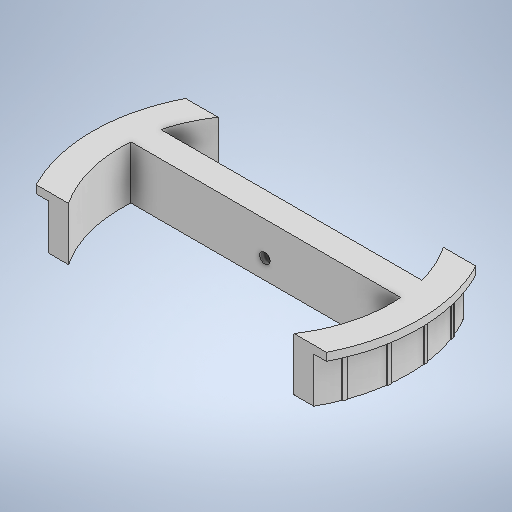
# Autodesk Inventor part: Part6
Saved by Autodesk Inventor 2025 (Build 290162010, 162A)
## iProperties
Created: 2024-07-08
Part Number: Part6
Material: Generic
Document SubType Name: Modeling
Designer: vncnt
Density: 1 g/cm^3
Appearance: Default
Author: vncnt
## iProperties of the stored document AQS_Mount_3DPrint.ipt
Created: 2024-07-08
Part Number: AQS_Mount_3DPrint
Material: Generic
Document SubType Name: Modeling
Designer: vncnt
Density: 1 g/cm^3
Appearance: Default
Author: vncnt
Autodesk Inventor part; units mm, degrees
ref_plane "YZ Plane" through (0, 0, 0) normal (1, 0, 0) x (0, 1, 0)
ref_plane "XZ Plane" through (0, 0, 0) normal (0, 1, 0) x (-1, 0, 0)
ref_plane "XY Plane" through (0, 0, 0) normal (0, 0, 1) x (1, 0, 0)
sketch "Sketch1" plane through (0, 0, 0) normal (0, 1, 0) x (-1, 0, 0)
  line L0 (33.8585, -6) -> (-33.8585, -6)
  line L1 (-34.295, -2.5) -> (34.295, -2.5)
  line L2 (0.5017, -38.45) -> (-0.4983, -38.45)
  line L3 (-0.4983, -38.45) -> (-0.4983, -38.85)
  line L4 (-0.4983, -38.85) -> (0.5017, -38.85)
  line L5 (0.5017, -38.85) -> (0.5017, -38.45)
  line L6 (0.5017, -38.45) -> (-0.4983, -38.85) construction
  line L7 (-0.4983, -38.45) -> (0.5017, -38.85) construction
  line L8 (9.6888, -37.2126) -> (8.7179, -37.452)
  line L9 (8.7179, -37.452) -> (8.8136, -37.8403)
  line L10 (8.8136, -37.8403) -> (9.7846, -37.601)
  line L11 (9.7846, -37.601) -> (9.6888, -37.2126)
  line L12 (18.3129, -33.8126) -> (17.4274, -34.2773)
  line L13 (17.4274, -34.2773) -> (17.6133, -34.6315)
  line L14 (17.6133, -34.6315) -> (18.4987, -34.1668)
  line L15 (18.4987, -34.1668) -> (18.3129, -33.8126)
  line L16 (25.8726, -28.4475) -> (25.1241, -29.1107)
  line L17 (25.1241, -29.1107) -> (25.3893, -29.4101)
  line L18 (25.3893, -29.4101) -> (26.1379, -28.7469)
  line L19 (26.1379, -28.7469) -> (25.8726, -28.4475)
  line L20 (31.9287, -21.4292) -> (31.3607, -22.2522)
  line L21 (31.3607, -22.2522) -> (31.6899, -22.4794)
  line L22 (31.6899, -22.4794) -> (32.2579, -21.6564)
  line L23 (32.2579, -21.6564) -> (31.9287, -21.4292)
  line L24 (36.1293, -13.1654) -> (35.7747, -14.1005)
  line L25 (35.7747, -14.1005) -> (36.1487, -14.2423)
  line L26 (36.1487, -14.2423) -> (36.5033, -13.3073)
  line L27 (36.5033, -13.3073) -> (36.1293, -13.1654)
  line L28 (38.2301, -4.1366) -> (38.1096, -5.1293)
  line L29 (38.1096, -5.1293) -> (38.5067, -5.1775)
  line L30 (38.5067, -5.1775) -> (38.6272, -4.1848)
  line L31 (38.6272, -4.1848) -> (38.2301, -4.1366)
  line L32 (38.1092, 5.1327) -> (38.2297, 4.14)
  line L33 (38.2297, 4.14) -> (38.6268, 4.1882)
  line L34 (38.6268, 4.1882) -> (38.5063, 5.1809)
  line L35 (38.5063, 5.1809) -> (38.1092, 5.1327)
  line L36 (35.7735, 14.1037) -> (36.1281, 13.1687)
  line L37 (36.1281, 13.1687) -> (36.5021, 13.3105)
  line L38 (36.5021, 13.3105) -> (36.1475, 14.2455)
  line L39 (36.1475, 14.2455) -> (35.7735, 14.1037)
  line L40 (31.3587, 22.255) -> (31.9268, 21.432)
  line L41 (31.9268, 21.432) -> (32.256, 21.6592)
  line L42 (32.256, 21.6592) -> (31.6879, 22.4822)
  line L43 (31.6879, 22.4822) -> (31.3587, 22.255)
  line L44 (25.1215, 29.1129) -> (25.87, 28.4498)
  line L45 (25.87, 28.4498) -> (26.1353, 28.7492)
  line L46 (26.1353, 28.7492) -> (25.3868, 29.4123)
  line L47 (25.3868, 29.4123) -> (25.1215, 29.1129)
  line L48 (17.4244, 34.2789) -> (18.3098, 33.8142)
  line L49 (18.3098, 33.8142) -> (18.4957, 34.1684)
  line L50 (18.4957, 34.1684) -> (17.6102, 34.6331)
  line L51 (17.6102, 34.6331) -> (17.4244, 34.2789)
  line L52 (8.7145, 37.4528) -> (9.6855, 37.2135)
  line L53 (9.6855, 37.2135) -> (9.7812, 37.6018)
  line L54 (9.7812, 37.6018) -> (8.8103, 37.8412)
  line L55 (8.8103, 37.8412) -> (8.7145, 37.4528)
  line L56 (-0.5017, 38.45) -> (0.4983, 38.45)
  line L57 (0.4983, 38.45) -> (0.4983, 38.85)
  line L58 (0.4983, 38.85) -> (-0.5017, 38.85)
  line L59 (-0.5017, 38.85) -> (-0.5017, 38.45)
  line L60 (-9.6888, 37.2126) -> (-8.7179, 37.452)
  line L61 (-8.7179, 37.452) -> (-8.8136, 37.8403)
  line L62 (-8.8136, 37.8403) -> (-9.7846, 37.601)
  line L63 (-9.7846, 37.601) -> (-9.6888, 37.2126)
  line L64 (-18.3129, 33.8126) -> (-17.4274, 34.2773)
  line L65 (-17.4274, 34.2773) -> (-17.6133, 34.6315)
  line L66 (-17.6133, 34.6315) -> (-18.4987, 34.1668)
  line L67 (-18.4987, 34.1668) -> (-18.3129, 33.8126)
  line L68 (-25.8726, 28.4475) -> (-25.1241, 29.1107)
  line L69 (-25.1241, 29.1107) -> (-25.3893, 29.4101)
  line L70 (-25.3893, 29.4101) -> (-26.1379, 28.7469)
  line L71 (-26.1379, 28.7469) -> (-25.8726, 28.4475)
  line L72 (-31.9287, 21.4292) -> (-31.3607, 22.2522)
  line L73 (-31.3607, 22.2522) -> (-31.6899, 22.4794)
  line L74 (-31.6899, 22.4794) -> (-32.2579, 21.6564)
  line L75 (-32.2579, 21.6564) -> (-31.9287, 21.4292)
  line L76 (-36.1293, 13.1654) -> (-35.7747, 14.1005)
  line L77 (-35.7747, 14.1005) -> (-36.1487, 14.2423)
  line L78 (-36.1487, 14.2423) -> (-36.5033, 13.3073)
  line L79 (-36.5033, 13.3073) -> (-36.1293, 13.1654)
  line L80 (-38.2301, 4.1366) -> (-38.1096, 5.1293)
  line L81 (-38.1096, 5.1293) -> (-38.5067, 5.1775)
  line L82 (-38.5067, 5.1775) -> (-38.6272, 4.1848)
  line L83 (-38.6272, 4.1848) -> (-38.2301, 4.1366)
  line L84 (-38.1092, -5.1327) -> (-38.2297, -4.14)
  line L85 (-38.2297, -4.14) -> (-38.6268, -4.1882)
  line L86 (-38.6268, -4.1882) -> (-38.5063, -5.1809)
  line L87 (-38.5063, -5.1809) -> (-38.1092, -5.1327)
  line L88 (-35.7735, -14.1037) -> (-36.1281, -13.1687)
  line L89 (-36.1281, -13.1687) -> (-36.5021, -13.3105)
  line L90 (-36.5021, -13.3105) -> (-36.1475, -14.2455)
  line L91 (-36.1475, -14.2455) -> (-35.7735, -14.1037)
  line L92 (-31.3587, -22.255) -> (-31.9268, -21.432)
  line L93 (-31.9268, -21.432) -> (-32.256, -21.6592)
  line L94 (-32.256, -21.6592) -> (-31.6879, -22.4822)
  line L95 (-31.6879, -22.4822) -> (-31.3587, -22.255)
  line L96 (-25.1215, -29.1129) -> (-25.87, -28.4498)
  line L97 (-25.87, -28.4498) -> (-26.1353, -28.7492)
  line L98 (-26.1353, -28.7492) -> (-25.3868, -29.4123)
  line L99 (-25.3868, -29.4123) -> (-25.1215, -29.1129)
  line L100 (-17.4244, -34.2789) -> (-18.3098, -33.8142)
  line L101 (-18.3098, -33.8142) -> (-18.4957, -34.1684)
  line L102 (-18.4957, -34.1684) -> (-17.6102, -34.6331)
  line L103 (-17.6102, -34.6331) -> (-17.4244, -34.2789)
  line L104 (-8.7145, -37.4528) -> (-9.6855, -37.2135)
  line L105 (-9.6855, -37.2135) -> (-9.7812, -37.6018)
  line L106 (-9.7812, -37.6018) -> (-8.8103, -37.8412)
  line L107 (-8.8103, -37.8412) -> (-8.7145, -37.4528)
  arc A0 (-33.6574, 19) -> (32.0907, -21.5409) centre (0, 0) ccw
  arc A1 (33.6574, -19) -> (33.6574, 19) centre (0, 0) ccw
  arc A2 (32.0887, 21.5438) -> (-32.0907, 21.5409) centre (0, 0) ccw
  line L108 (36.1642, -3.8857) -> (36.1642, -3.8892)
  line L109 (36.1642, -4.8931) -> (36.1642, -4.8965)
  line L110 (-34.9312, -4.7468) -> (-34.9312, -4.7433)
  line L111 (-34.9312, -3.7395) -> (-34.9312, -3.736)
  line L112 (33.6574, -19) -> (28.66, -19)
  line L113 (-28.66, -19) -> (-33.6574, -19)
  line L114 (-33.6574, 19) -> (-28.66, 19)
  line L115 (28.66, 19) -> (33.6574, 19)
  arc A3 (28.66, -19) -> (33.8585, -6) centre (0, 0) ccw
  arc A4 (34.295, -2.5) -> (28.66, 19) centre (0, 0) ccw
  arc A5 (-28.66, 19) -> (-34.295, -2.5) centre (0, 0) ccw
  arc A6 (-33.8585, -6) -> (-28.66, -19) centre (0, 0) ccw
  point P0 (0.0017, -38.65)
  point P1 (35.9587, -14.1702)
  point P2 (36.3132, -13.2352)
  point P3 (38.3049, -5.153)
  point P4 (38.4254, -4.1603)
  point P5 (38.4251, 4.1637)
  point P6 (38.3045, 5.1564)
  point P7 (36.3121, 13.2384)
  point P8 (35.9574, 14.1734)
  point P9 (-35.9587, 14.1702)
  point P10 (-36.3132, 13.2352)
  point P11 (-38.3049, 5.153)
  point P12 (-38.4254, 4.1603)
  point P13 (-38.4251, -4.1637)
  point P14 (-38.3045, -5.1564)
  point P15 (-36.3121, -13.2384)
  point P16 (-35.9574, -14.1734)
  dimension "d2" = 2.5
  dimension "d3" = 3.5
  dimension "d10" = 1
  dimension "d11" = 0.4
  dimension "d14" = 360
  dimension "d18" = 38.65
  dimension "d19" = 4.9974
  constraints: 232 end point, 16 point on circle, 11 parallel, 11 point on line, 7 centre point, 4 horizontal, 3 perpendicular, 2 midpoint, 1 coincident, 209 other
  measures "d2" distance from line of L1 point (0, 0)
  measures "d3" distance between parallel lines of L1 L0
  measures "d10" distance of L4.end L3.end
  measures "d11" distance of L3.end L2.end
  measures "d18" radius of A0
  measures "d19" distance of L113.start L113.end
extrude "Extrusion1" add sketch "Sketch1" along normal blind 11.5 contours L0 A6 L113 A0 L91 L88 L89 L87 L84 L85 L83 L80 L81 L79 L76 L77 L114 A5 L1 A4 L115 A1 L39 L36 L37 L35 L32 L33 L31 L28 L29 L27 L24 L25 L112 A3 | A1 L27 L26 L25 | L25 L24 L27 A1 | A0 L89 L88 L91 | L91 L90 L89 A0 | A1 L31 L30 L29 | L29 L28 L31 A1 | A0 L85 L84 L87 | L87 L86 L85 A0 | A1 L35 L34 L33 | L33 L32 L35 A1 | A0 L81 L80 L83 | L83 L82 L81 A0 | A1 L39 L38 L37 | L37 L36 L39 A1 | A0 L77 L76 L79 | L79 L78 L77 A0
sketch "Sketch2" plane through (0, 11.5, 0) normal (0, 1, 0) x (1, 0, 0)
  arc A0 (33.8585, 6) -> (28.66, 19) centre (0, 0) ccw projected
  line L0 (34.295, 2.5) -> (-34.295, 2.5)
  line L1 (-3.804, 9) -> (7.0469, 9)
  line L2 (33.1873, 9) -> (-33.1873, 9)
  line L3 (-28.66, 19) -> (-33.6574, 19) projected
  line L4 (-33.6574, -19) -> (-28.66, -19) projected
  line L5 (-28.66, -19) -> (-36.8951, -19)
  arc A1 (-34.295, 2.5) -> (-28.66, -19) centre (0, 0) ccw
  arc A2 (28.66, -19) -> (34.295, 2.5) centre (0, 0) ccw
  arc A3 (36.8951, -19) -> (36.8951, 19) centre (0, 0) ccw
  arc A4 (-36.8951, 19) -> (-36.8951, -19) centre (0, 0) ccw
  arc A5 (33.1873, 9) -> (28.66, 19) centre (0, 0) ccw
  arc A6 (-28.66, 19) -> (-33.1873, 9) centre (0, 0) ccw
  line L6 (36.8951, 19) -> (28.66, 19)
  line L7 (-28.66, 19) -> (-36.8951, 19)
  line L8 (-31.7819, -19) -> (-28.66, -19)
  line L9 (28.66, -19) -> (36.8951, -19)
  line L10 (-30.5962, 19) -> (-28.66, 19)
  line L11 (28.66, 19) -> (36.8951, 19)
  point P0 (28.66, 19)
  point P1 (7.0469, 9)
  dimension "d24" = 41.5
  dimension "d25" = 6.5
  constraints: 20 end point, 13 point on circle, 6 centre point, 4 horizontal, 2 coincident, 2 collinear, 2 point on line
  measures "d24" radius of A4
  measures "d25" distance between parallel lines of L0 L2
extrude "Extrusion2" add sketch "Sketch2" along normal blind 2
sketch "Sketch3" plane through (-34.295, 0, -2.5) normal (0, 0, 1) x (1, 0, 0)
  line L0 (0, 13.5) -> (68.59, 13.5) projected
  line L1 (0, 0) -> (0, 13.5) projected
  point P0 (34.295, 0)
  point P1 (34.0614, 4.8894)
  dimension "d28" = 8.6106
  dimension "d29" = 34.0614
  measures "d28" distance from line of L0 point (34.061, 4.889)
  measures "d29" distance from line of L1 point (34.061, 4.889)
hole "Hole1" at (-0.2336, 4.8894, -2.5) direction (0, 0, -1) diameter 2.6416 depth 10.979 thread size "6-32 UNC" class "2B" standard "ANSI Unified Screw Threads"
body "Solid1"
